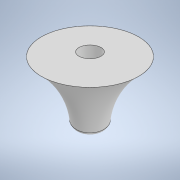
# Autodesk Inventor part: knob_bottom
Saved by Autodesk Inventor 2022 (Build 260153000, 153)
## iProperties
Created: 2022-06-07
Part Number: knob_bottom
Material: Generic
Document SubType Name: Modeling
Designer: Jacob
Density: 1 g/cm^3
Appearance: Default
Author: Jacob
Autodesk Inventor part; units mm, degrees
ref_plane "YZ Plane" through (0, 0, 0) normal (1, 0, 0) x (0, 1, 0)
ref_plane "XZ Plane" through (0, 0, 0) normal (0, 1, 0) x (-1, 0, 0)
ref_plane "XY Plane" through (0, 0, 0) normal (0, 0, 1) x (1, 0, 0)
sketch "Sketch1" plane through (0, 0, 0) normal (0, 0, 1) x (1, 0, 0)
  line L0 (0, 0) -> (0, 7.8365) construction
  line L1 (1.275, 0) -> (3.775, 0)
  line L2 (1.275, 0) -> (1.275, 8)
  line L3 (1.275, 8) -> (2.3, 8)
  line L4 (2.3, 8) -> (2.3, 15)
  line L5 (2.3, 15) -> (10, 15)
  arc A0 (10, 15) -> (3.775, 0) centre (24.9598, 0) ccw
  dimension "d0" = 1.275
  dimension "d1" = 15
  dimension "d2" = 8
  dimension "d3" = 2.3
  dimension "d4" = 10
  dimension "d5" = 2.5
  constraints: 12 end point, 2 horizontal, 2 perpendicular, 2 point on circle, 2 vertical, 1 centre point, 1 line through centre, 1 point on line
  measures "d0" distance between parallel lines of L0 L2
  measures "d1" distance between parallel lines of L5 L1
  measures "d2" distance of L1.start L2.end
  measures "d3" distance between parallel lines of L0 L4
  measures "d4" distance from line of L0 L5.end
  measures "d5" distance of L1.start L1.end
revolve "Revolution1" add sketch "Sketch1" angle 360 about axis through (0, 0, 0) along (0, 1, 0)
fillet "Fillet1" radius 1 1 edges at (-3.775, 0, 0)
sketch "Sketch2" plane through (0, 15, 0) normal (0, 1, 0) x (1, 0, 0)
  circle A0 centre (0, 0) radius 2.3 projected
  circle A1 centre (0, 0) radius 10 projected
body "Solid1"
